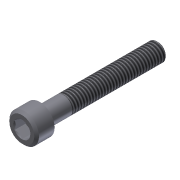
# Autodesk Inventor part: 10-32 x1000
Saved by Autodesk Inventor 2013 (Build 170138000, 138)
## iProperties
Created: 2011-07-11
Part Number: 10-32 x1000
Document SubType Name: Modeling
Designer: Dan Niemitalo
Density: 7.85 g/cm^3
Material: Steel
Mass: 6.04932 g
Surface Area: 7.31231 cm^2
Volume: 0.770614 cm^3
Author: Dan Niemitalo
Autodesk Inventor part; units mm, degrees
ref_plane "YZ Plane" through (0, 0, 0) normal (1, 0, 0) x (0, 1, 0)
ref_plane "XZ Plane" through (0, 0, 0) normal (0, 1, 0) x (-1, 0, 0)
ref_plane "XY Plane" through (0, 0, 0) normal (0, 0, 1) x (1, 0, 0)
sketch "Sketch1" plane through (0, 0, 0) normal (0, 0, 1) x (1, 0, 0)
  circle A0 centre (0, 0) radius 3.9624
  dimension "cap_diam" = 7.9248
  constraints: 1 centre point, 1 coincident
  measures "cap_diam" diameter of A0
extrude "Extrusion1" add sketch "Sketch1" along normal blind 4.826
sketch "Sketch2" plane through (0, 0, 0) normal (0, 0, -1) x (-1, 0, 0)
  circle A0 centre (0, 0) radius 3.9624 projected
  circle A1 centre (0, 0) radius 2.413
  dimension "thread_diam" = 4.826
  constraints: 1 centre point, 1 coincident
  measures "thread_diam" diameter of A1
extrude "Extrusion2" add sketch "Sketch2" along normal blind 31.75 contours A1
thread "Thread1" size "10-32 UNF" class "2A" standard "ANSI Unified Screw Threads" length 25.4
chamfer "Chamfer1" distance 0.4064 angle 45 1 edges at (2.413, 0, -31.75)
chamfer "Chamfer2" distance 0.635 angle 45 1 edges at (-3.9624, 0, 4.826)
sketch "Sketch4" plane through (0, 0, 4.826) normal (0, 0, 1) x (1, 0, 0)
  circle A0 centre (0, 0) radius 3.3274 projected
  circle A1 centre (0, 0) radius 1.9844
  dimension "d21" = 3.9688
  constraints: 1 centre point, 1 coincident
  measures "d21" diameter of A1
extrude "Extrusion4" cut sketch "Sketch4" against normal blind 0.3048 contours A1
chamfer "Chamfer3" distance 0.3048 angle 45 1 edges at (-1.9844, 0, 4.826)
sketch "Sketch5" plane through (0, 0, 4.826) normal (0, 0, 1) x (1, 0, 0)
  circle A0 centre (0, 0) radius 2.2892 construction
  line L0 (0, 2.2914) -> (1.9844, 1.1457)
  line L1 (1.9844, 1.1457) -> (1.9844, -1.1457)
  line L2 (1.9844, -1.1457) -> (0, -2.2914)
  line L3 (0, -2.2914) -> (-1.9844, -1.1457)
  line L4 (-1.9844, -1.1457) -> (-1.9844, 1.1457)
  line L5 (-1.9844, 1.1457) -> (0, 2.2914)
  dimension "d27" = 3.9688
  constraints: 12 end point, 1 coincident, 1 vertical, 13 other
  measures "d27" distance between parallel lines of L4 L1
extrude "Extrusion5" cut sketch "Sketch5" against normal blind 2.9718
equation "\"d21\" = hex_diam"
equation "\"hex_diam\" = 3.96875"
body "Solid1"
